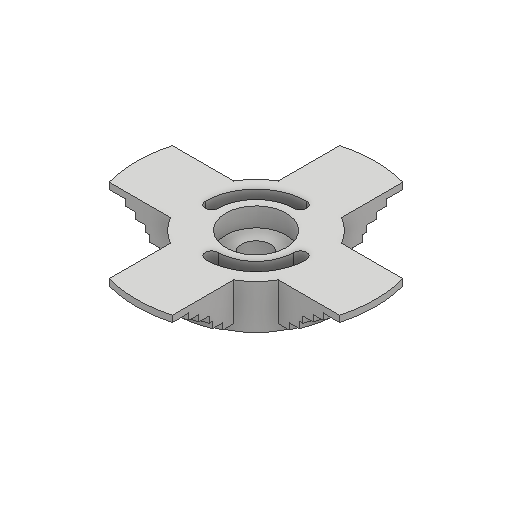
# Autodesk Inventor part: 3DP_ABS_Filament_Spool_Mount_Bearing_Block
Saved by Autodesk Inventor 2026.1 (Build 301233000, 233)
## iProperties
Created: 2015-12-11
Part Number: 3DP_ABS_Filament_Spool_Mount_Bearing_Block
Material: Ogólny
Document SubType Name: Modeling
Designer: Andrzej
Density: 1 g/cm^3
Appearance: Domyślna
Author: Andrzej
Autodesk Inventor part; units mm, degrees
ref_plane "YZ Plane" through (0, 0, 0) normal (1, 0, 0) x (0, 1, 0)
ref_plane "XZ Plane" through (0, 0, 0) normal (0, 1, 0) x (-1, 0, 0)
ref_plane "XY Plane" through (0, 0, 0) normal (0, 0, 1) x (1, 0, 0)
sketch "Szkic1" plane through (0, 0, 0) normal (0, 0, 1) x (1, 0, 0)
  line L0 (-20.4343, -10) -> (-41.564, -10)
  line L1 (-20.4343, 10) -> (-41.564, 10)
  line L2 (-10, -20.4343) -> (-10, -41.564)
  line L3 (10, -20.4343) -> (10, -41.564)
  line L4 (20.4343, -10) -> (41.564, -10)
  line L5 (20.4343, 10) -> (41.564, 10)
  line L6 (10, 20.4343) -> (10, 41.564)
  line L7 (-10, 20.4343) -> (-10, 41.564)
  arc A0 (-36.4014, 10) -> (-36.4014, -10) centre (0, 0) ccw
  arc A1 (-31.1859, 10) -> (-31.1859, -10) centre (0, 0) ccw
  arc A2 (-28.019, 10) -> (-28.019, -10) centre (0, 0) ccw
  arc A3 (-24.8105, 10) -> (-24.8105, -10) centre (0, 0) ccw
  arc A4 (-23.7289, 10) -> (-23.7289, -10) centre (0, 0) ccw
  arc A5 (-20.4343, 10) -> (-20.4343, -10) centre (0, 0) ccw
  arc A6 (-41.564, 10) -> (-41.564, -10) centre (0, 0) ccw
  arc A7 (-10, -20.4343) -> (10, -20.4343) centre (0, 0) ccw
  arc A8 (-10, -23.7289) -> (10, -23.7289) centre (0, 0) ccw
  arc A9 (-10, -24.8105) -> (10, -24.8105) centre (0, 0) ccw
  arc A10 (-10, -28.019) -> (10, -28.019) centre (0, 0) ccw
  arc A11 (-10, -31.1859) -> (10, -31.1859) centre (0, 0) ccw
  arc A12 (-10, -36.4014) -> (10, -36.4014) centre (0, 0) ccw
  arc A13 (-10, -41.564) -> (10, -41.564) centre (0, 0) ccw
  arc A14 (20.4343, -10) -> (20.4343, 10) centre (0, 0) ccw
  arc A15 (10, 20.4343) -> (-10, 20.4343) centre (0, 0) ccw
  arc A16 (23.7289, -10) -> (23.7289, 10) centre (0, 0) ccw
  arc A17 (10, 23.7289) -> (-10, 23.7289) centre (0, 0) ccw
  arc A18 (24.8105, -10) -> (24.8105, 10) centre (0, 0) ccw
  arc A19 (10, 24.8105) -> (-10, 24.8105) centre (0, 0) ccw
  arc A20 (28.019, -10) -> (28.019, 10) centre (0, 0) ccw
  arc A21 (10, 28.019) -> (-10, 28.019) centre (0, 0) ccw
  arc A22 (31.1859, -10) -> (31.1859, 10) centre (0, 0) ccw
  arc A23 (10, 31.1859) -> (-10, 31.1859) centre (0, 0) ccw
  arc A24 (36.4014, -10) -> (36.4014, 10) centre (0, 0) ccw
  arc A25 (10, 36.4014) -> (-10, 36.4014) centre (0, 0) ccw
  arc A26 (41.564, -10) -> (41.564, 10) centre (0, 0) ccw
  arc A27 (10, 41.564) -> (-10, 41.564) centre (0, 0) ccw
  circle A28 centre (0, 0) radius 4.5
  circle A29 centre (0, 0) radius 19.75
  line L8 (10, 20.4343) -> (10, 17.0312)
  line L9 (-10, 20.4343) -> (-10, 17.0312)
  line L10 (10, -20.4343) -> (10, -17.0312)
  line L11 (-20.4343, -10) -> (-17.0312, -10)
  line L12 (-20.4343, 10) -> (-17.0312, 10)
  line L13 (-10, -17.0312) -> (-10, -20.4343)
  line L14 (20.4343, 10) -> (17.0312, 10)
  line L15 (20.4343, -10) -> (17.0312, -10)
  line L16 (0, -4.5265) -> (0, 3.8342)
  line L17 (3.7027, 0) -> (-4.6541, 0)
  arc A30 (0, -14) -> (14, 0) centre (0, 0) ccw construction
  arc A31 (0, -16.5) -> (16.5, 0) centre (0, 0) ccw
  arc A32 (0, -11.5) -> (11.5, 0) centre (0, 0) ccw
  arc A33 (0, -11.5) -> (0, -16.5) centre (0, -14) ccw
  arc A34 (16.5, 0) -> (11.5, 0) centre (14, 0) ccw
  arc A35 (0, 14) -> (-14, 0) centre (0, 0) ccw construction
  arc A36 (0, 16.5) -> (-16.5, 0) centre (0, 0) ccw
  arc A37 (0, 11.5) -> (-11.5, 0) centre (0, 0) ccw
  arc A38 (0, 11.5) -> (0, 16.5) centre (0, 14) ccw
  arc A39 (-16.5, 0) -> (-11.5, 0) centre (-14, 0) ccw
  arc A40 (0, -12) -> (12, 0) centre (0, 0) ccw
  arc A41 (0, -12) -> (0, -16) centre (0, -14) ccw
  arc A42 (0, -16) -> (16, 0) centre (0, 0) ccw
  arc A43 (16, 0) -> (12, 0) centre (14, 0) ccw
  arc A44 (0, 12) -> (-12, 0) centre (0, 0) ccw
  arc A45 (0, 12) -> (0, 16) centre (0, 14) ccw
  arc A46 (0, 16) -> (-16, 0) centre (0, 0) ccw
  arc A47 (-16, 0) -> (-12, 0) centre (-14, 0) ccw
  point P0 (10, -17.0312)
  point P1 (-10, -17.0312)
  point P2 (-10, 17.0312)
  dimension "d62" = 22.75
  dimension "d14" = 9
  dimension "d42" = 14
  dimension "d43" = 14
  dimension "d44" = 14
  dimension "d45" = 14
  dimension "d47" = 5
  dimension "d48" = 5
  dimension "d57" = 0.5
  dimension "d58" = 0.5
  constraints: 40 point on line, 36 end point, 36 point on circle, 19 centre point, 14 horizontal alignment, 14 vertical alignment, 8 tangent, 4 horizontal, 2 coincident, 2 vertical, 1 collinear, 73 other
  measures "d14" diameter of A28
  measures "d42" distance from line of L16 A30.end
  measures "d43" distance from line of L17 A30.start
  measures "d44" distance from line of A35.start L17
  measures "d45" distance from line of L16 A35.end
  measures "d47" diameter of A34
  measures "d48" diameter of A38
  measures "d57" radial gap between concentric circles of A34 A43
  measures "d58" radial gap between concentric circles of A37 A44
extrude "Wyciągnięcie proste2" add sketch "Szkic1" along normal blind 14 contours L0 A4 L1 A5 | A5 L12 A29 L11 | L0 A3 L1 A4 | A29 | L0 A2 L1 A3 | A29 L10 A7 L13 | L0 A1 L1 A2 | L9 A15 L8 A29 | A7 L3 A8 L2 | L0 A0 L1 A1 | L7 A17 L6 A15 | A29 L14 A14 L15 | A8 L3 A9 L2 | L0 A6 L1 A0 | L7 A19 L6 A17 | A14 L5 A16 L4 | A9 L3 A10 L2 | L7 A21 L6 A19 | A16 L5 A18 L4 | A10 L3 A11 L2 | L7 A23 L6 A21 | A18 L5 A20 L4 | A11 L3 A12 L2 | L7 A25 L6 A23 | A20 L5 A22 L4 | A12 L3 A13 L2 | L7 A27 L6 A25 | A22 L5 A24 L4 | A24 L5 A26 L4 | A33 A32 A34 A31 | A38 A37 A39 A36 | A40 A43 A42 A41 | A44 A47 A46 A45
extrude "Wyciągnięcie proste3" cut sketch "Szkic1" along normal blind 2 contours A5 L12 A29 L11 | A29 L10 A7 L13 | L9 A15 L8 A29 | A29 L14 A14 L15
extrude "Wyciągnięcie proste4" cut sketch "Szkic1" along normal blind 4 contours L0 A4 L1 A5 | A7 L3 A8 L2 | L7 A17 L6 A15 | A14 L5 A16 L4
extrude "Wyciągnięcie proste5" cut sketch "Szkic1" along normal blind 6 contours L0 A3 L1 A4 | A8 L3 A9 L2 | L7 A19 L6 A17 | A16 L5 A18 L4
extrude "Wyciągnięcie proste6" cut sketch "Szkic1" along normal blind 8 contours L0 A2 L1 A3 | A9 L3 A10 L2 | L7 A21 L6 A19 | A18 L5 A20 L4
extrude "Wyciągnięcie proste7" cut sketch "Szkic1" along normal blind 10 contours L0 A1 L1 A2 | A10 L3 A11 L2 | L7 A23 L6 A21 | A20 L5 A22 L4
extrude "Wyciągnięcie proste8" cut sketch "Szkic1" along normal blind 12 contours L0 A0 L1 A1 | A11 L3 A12 L2 | L7 A25 L6 A23 | A22 L5 A24 L4
extrude "Wyciągnięcie proste9" cut sketch "Szkic1" along normal blind 15 contours L0 A6 L1 A0 | A12 L3 A13 L2 | L7 A27 L6 A25 | A24 L5 A26 L4
sketch "Szkic2" plane through (0, 0, 14) normal (0, 0, 1) x (1, 0, 0)
  circle A0 centre (0, 0) radius 4.5 projected
  line L0 (10, -36.4014) -> (10, -17.0312) projected
  arc A1 (10, -17.0312) -> (17.0312, -10) centre (0, 0) ccw projected
  line L1 (17.0312, -10) -> (36.4014, -10) projected
  line L2 (36.4014, 10) -> (17.0312, 10) projected
  arc A2 (17.0312, 10) -> (10, 17.0312) centre (0, 0) ccw projected
  line L3 (10, 17.0312) -> (10, 36.4014) projected
  line L4 (-10, 36.4014) -> (-10, 17.0312) projected
  arc A3 (-10, 17.0312) -> (-17.0312, 10) centre (0, 0) ccw projected
  line L5 (-17.0312, 10) -> (-36.4014, 10) projected
  line L6 (-36.4014, -10) -> (-17.0312, -10) projected
  arc A4 (-17.0312, -10) -> (-10, -17.0312) centre (0, 0) ccw projected
  line L7 (-10, -17.0312) -> (-10, -36.4014) projected
  circle A5 centre (0, 0) radius 9.5
  arc A6 (36.4014, -10) -> (36.4014, 10) centre (0, 0) ccw projected
  arc A7 (10, 36.4014) -> (-10, 36.4014) centre (0, 0) ccw projected
  arc A8 (-36.4014, 10) -> (-36.4014, -10) centre (0, 0) ccw projected
  arc A9 (-10, -36.4014) -> (10, -36.4014) centre (0, 0) ccw projected
  dimension "d33" = 19
  constraints: 1 centre point
  measures "d33" diameter of A5
extrude "Wyciągnięcie proste10" cut sketch "Szkic2" against normal blind 6 contours A5
chamfer "Faza2" distance 1 angle 45 1 edges at (-4.5, 0, 0)
extrude "Wyciągnięcie proste12" cut sketch "Szkic1" along normal blind 17 contours A40 A43 A42 A41 | A44 A47 A46 A45
